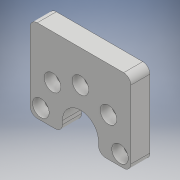
# Autodesk Inventor part: elbow_protection
Saved by Autodesk Inventor 2018 (Build 220112000, 112)
## iProperties
Created: 2018-04-22
Part Number: elbow_protection
Material: Generic
Document SubType Name: Modeling
Designer: medrimonia
Density: 1 g/cm^3
Appearance: Default
Vendor: Rhoban
Mass: 2.70718 g
Surface Area: 19.7582 cm^2
Volume: 2.70718 cm^3
Author: medrimonia
Autodesk Inventor part; units mm, degrees
ref_plane "YZ Plane" through (0, 0, 0) normal (1, 0, 0) x (0, 1, 0)
ref_plane "XZ Plane" through (0, 0, 0) normal (0, 1, 0) x (-1, 0, 0)
ref_plane "XY Plane" through (0, 0, 0) normal (0, 0, 1) x (1, 0, 0)
sketch "Sketch1" plane through (0, 0, 0) normal (0, 1, 0) x (-1, 0, 0)
  line L0 (14, 0) -> (-14, 0) construction
  line L1 (-14, 0) -> (-14, 20)
  line L2 (-14, 20) -> (14, 20)
  line L3 (14, 20) -> (14, 0)
  circle A0 centre (0, 0) radius 5
  line L4 (14, 0) -> (14, -3)
  line L5 (14, -3) -> (4, -3)
  line L6 (-14, -3) -> (-14, 0)
  line L7 (9.8995, 9.8995) -> (-9.8995, -9.8995) construction
  line L8 (0, 14) -> (0, -14) construction
  line L9 (-9.8995, 9.8995) -> (9.8995, -9.8995) construction
  line L10 (-14, 0) -> (14, 0) construction
  line L11 (-4, -3) -> (-14, -3)
  line L12 (4, -3) -> (-4, -3) construction
  line L13 (5, 0) -> (5, -1)
  line L14 (-5, 0) -> (-5, -1)
  arc A1 (-7, -3) -> (-5, -1) centre (-7, -1) ccw
  arc A2 (5, -1) -> (7, -3) centre (7, -1) ccw
  point P0 (11, 0)
  point P1 (7.7782, 7.7782)
  point P2 (0, 11)
  point P3 (-7.7782, 7.7782)
  point P4 (-11, 0)
  dimension "d0" = 28
  dimension "d1" = 10
  dimension "d2" = 20
  dimension "d3" = 3
  dimension "d4" = 11
  dimension "d7" = 180
  dimension "d20" = 1
  constraints: 30 end point, 8 point on circle, 8 point on line, 6 perpendicular, 6 tangent, 3 centre point, 3 parallel, 2 coincident, 1 collinear, 1 horizontal, 1 midpoint, 1 vertical, 21 other
  measures "d0" distance of L0.start L0.end
  measures "d1" diameter of A0
  measures "d2" distance between parallel lines of L2 L0
  measures "d3" distance between parallel lines of L0 L5
  measures "d4" distance of point (0, 0) point (11, 0)
  measures "d20" distance of L14.start L14.end
extrude "Extrusion1" add sketch "Sketch1" along normal blind 5.3 contours L1 L2 L3 L4 L5 A2 L13 A0 L14 A1 L11 L6
hole "Hole1" at (-11, 0, 0) at (-7.7782, 0, 7.7782) at (0, 0, 11) at (7.7782, 0, 7.7782) at (11, 0, 0) direction (0, 1, 0) diameter 2.5 end through all counterbore diameter 4.6 counterbore depth 3.1
fillet "Fillet2" radius 2 4 edges at (-14, 2.65, -3) (-14, 2.65, 20) (14, 2.65, 20) (14, 2.65, -3)
equation "\"d9\" = teflon_thickness"
equation "\"d13\" = trace_radius"
equation "\"d14\" = trace_depth"
equation "\"teflon_thickness\" = 5.3"
equation "\"trace_radius\" = 4.6"
equation "\"trace_depth\" = 3.1"
body "Solid1"
